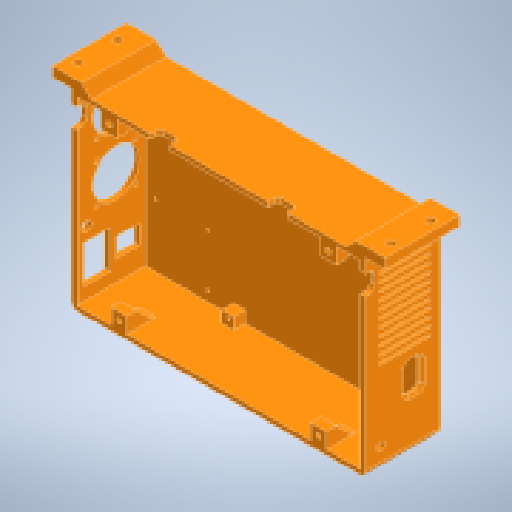
# Autodesk Inventor part: electronic_box
Saved by Autodesk Inventor 2024.1 (Build 281209000, 209)
## iProperties
Created: 2023-10-17
Part Number: electronic_box
Material: Generic
Document SubType Name: Modeling
Designer: l1534
Density: 1 g/cm^3
Appearance: Orange
Author: l1534
Autodesk Inventor part; units mm, degrees
ref_plane "YZ Plane" through (0, 0, 0) normal (1, 0, 0) x (0, 1, 0)
ref_plane "XZ Plane" through (0, 0, 0) normal (0, 1, 0) x (-1, 0, 0)
ref_plane "XY Plane" through (0, 0, 0) normal (0, 0, 1) x (1, 0, 0)
sketch "Sketch1" plane through (0, 0, 0) normal (0, 0, 1) x (1, 0, 0)
  line L0 (-76.6473, 17.8798) -> (73.3527, 17.8798)
  line L1 (73.3527, 17.8798) -> (73.3527, -79.3702)
  line L2 (73.3527, -79.3702) -> (-76.6473, -79.3702)
  line L3 (-76.6473, -79.3702) -> (-76.6473, 17.8798)
  point P0 (0, 0)
  dimension "d0" = 97.25
  dimension "d1" = 150
  constraints: 8 end point, 2 parallel, 1 horizontal, 1 perpendicular
  measures "d0" distance of L0.end L1.end
  measures "d1" distance of L1.end L2.end
extrude "Extrusion1" add sketch "Sketch1" along normal blind 38
sketch "Sketch2" plane through (0, 0, 38) normal (0, 0, 1) x (1, 0, 0)
  line L0 (-74.1473, 15.3798) -> (70.8527, 15.3798)
  line L1 (70.8527, 15.3798) -> (70.8527, -76.8702)
  line L2 (70.8527, -76.8702) -> (-74.1473, -76.8702)
  line L3 (-74.1473, -76.8702) -> (-74.1473, 15.3798)
  line L4 (73.3527, 17.8798) -> (-76.6473, 17.8798) projected
  line L5 (73.3527, -79.3702) -> (73.3527, 17.8798) projected
  line L6 (-76.6473, -79.3702) -> (73.3527, -79.3702) projected
  line L7 (-76.6473, 17.8798) -> (-76.6473, -79.3702) projected
  point P0 (0, 0)
  dimension "d4" = 2.5
  dimension "d5" = 2.5
  dimension "d6" = 2.5
  dimension "d7" = 2.5
  constraints: 8 end point, 2 parallel, 1 horizontal, 1 perpendicular
  measures "d4" distance between parallel lines of L4 L0
  measures "d5" distance between parallel lines of L5 L1
  measures "d6" distance between parallel lines of L6 L2
  measures "d7" distance between parallel lines of L7 L3
extrude "Extrusion2" cut sketch "Sketch2" against normal blind 35 contours L0 L1 L2 L3
sketch "Sketch3" plane through (0, 0, 3) normal (0, 0, 1) x (1, 0, 0)
  line L0 (-74.1473, 15.3798) -> (70.8527, 15.3798) projected
  line L1 (70.8527, 15.3798) -> (64.8527, 15.3798)
  line L2 (64.8527, 15.3798) -> (64.8527, 9.3798)
  line L3 (64.8527, 9.3798) -> (70.8527, 9.3798)
  line L4 (70.8527, 9.3798) -> (70.8527, 15.3798)
  line L5 (70.8527, -76.8702) -> (-74.1473, -76.8702) projected
  line L6 (70.8527, -76.8702) -> (64.8527, -76.8702)
  line L7 (64.8527, -76.8702) -> (64.8527, -70.8702)
  line L8 (64.8527, -70.8702) -> (70.8527, -70.8702)
  line L9 (70.8527, -70.8702) -> (70.8527, -76.8702)
  line L10 (-29.1473, -76.8702) -> (-23.1473, -76.8702)
  line L11 (-23.1473, -76.8702) -> (-23.1473, -70.8702)
  line L12 (-23.1473, -70.8702) -> (-29.1473, -70.8702)
  line L13 (-29.1473, -70.8702) -> (-29.1473, -76.8702)
  line L14 (-29.1473, 15.3798) -> (-23.1473, 15.3798)
  line L15 (-23.1473, 15.3798) -> (-23.1473, 9.3798)
  line L16 (-23.1473, 9.3798) -> (-29.1473, 9.3798)
  line L17 (-29.1473, 9.3798) -> (-29.1473, 15.3798)
  point P0 (0, 0)
  point P1 (64.8527, -73.8702)
  point P2 (-23.1473, -73.8702)
  point P3 (-23.1473, 15.3798)
  point P4 (-29.1473, 15.3798)
  dimension "d10" = 6
  dimension "d11" = 6
  dimension "d12" = 6
  dimension "d13" = 6
  dimension "d14" = 6
  dimension "d15" = 6
  dimension "d16" = 6
  dimension "d17" = 6
  dimension "d18" = 88
  dimension "d19" = 88
  constraints: 32 end point, 8 parallel, 4 horizontal, 4 perpendicular, 2 midpoint, 2 point on line
  measures "d10" distance of L1.end L2.end
  measures "d11" distance of L2.end L3.end
  measures "d12" distance of L7.end L8.end
  measures "d13" distance of L6.end L7.end
  measures "d14" distance of L10.end L11.end
  measures "d15" distance of L11.end L12.end
  measures "d16" distance of L15.end L16.end
  measures "d17" distance of L14.end L15.end
  measures "d18" distance between parallel lines of L2 L15
  measures "d19" distance of point (64.853, -73.87) point (-23.147, -73.87)
extrude "Extrusion3" add sketch "Sketch3" along normal blind 6
sketch "Sketch4" plane through (0, 0, 9) normal (0, 0, 1) x (1, 0, 0)
  circle A0 centre (66.8527, -73.1202) radius 0.9
  line L0 (70.8527, -76.8702) -> (-74.1473, -76.8702) projected
  line L1 (70.8527, 15.3798) -> (70.8527, -76.8702) projected
  point P0 (0, 0)
  dimension "d22" = 1.8
  dimension "d23" = 3.75
  dimension "d24" = 4
  constraints: 1 centre point
  measures "d22" diameter of A0
  measures "d23" distance from line of L0 A0.centre
  measures "d24" distance from line of L1 A0.centre
extrude "Extrusion4" cut sketch "Sketch4" against normal through all
sketch "Sketch5" plane through (0, 0, 9) normal (0, 0, 1) x (1, 0, 0)
  circle A0 centre (66.8527, 11.3798) radius 0.9
  line L0 (64.8527, 9.3798) -> (70.8527, 9.3798) projected
  line L1 (64.8527, 15.3798) -> (64.8527, 9.3798) projected
  point P0 (0, 0)
  dimension "d27" = 1.8
  dimension "d28" = 2
  dimension "d29" = 2
  constraints: 1 centre point
  measures "d27" diameter of A0
  measures "d28" distance from line of L0 A0.centre
  measures "d29" distance from line of L1 A0.centre
extrude "Extrusion5" cut sketch "Sketch5" against normal through all
sketch "Sketch6" plane through (0, 0, 9) normal (0, 0, 1) x (1, 0, 0)
  circle A0 centre (-25.6473, 11.3798) radius 0.9
  circle A1 centre (-25.6473, -73.1202) radius 0.9
  line L0 (-23.1473, 9.3798) -> (-23.1473, 15.3798) projected
  line L1 (-29.1473, 9.3798) -> (-23.1473, 9.3798) projected
  line L2 (-23.1473, -76.8702) -> (-23.1473, -70.8702) projected
  line L3 (-23.1473, -70.8702) -> (-29.1473, -70.8702) projected
  point P0 (0, 0)
  dimension "d32" = 1.8
  dimension "d33" = 1.8
  dimension "d34" = 2.5
  dimension "d35" = 2
  dimension "d36" = 2.5
  dimension "d37" = 2.25
  constraints: 2 centre point
  measures "d32" diameter of A1
  measures "d33" diameter of A0
  measures "d34" distance from line of L0 A0.centre
  measures "d35" distance from line of L1 A0.centre
  measures "d36" distance from line of L2 A1.centre
  measures "d37" distance from line of L3 A1.centre
extrude "Extrusion6" cut sketch "Sketch6" against normal through all
sketch "Sketch7" plane through (70.8527, -76.8702, 38) normal (-1, 0, 0) x (0, 0, 1)
  line L0 (-20.5, 37.5) -> (-28.5, 37.5)
  line L1 (-28.5, 37.5) -> (-28.5, 22.5)
  line L2 (-28.5, 22.5) -> (-20.5, 22.5)
  line L3 (-20.5, 22.5) -> (-20.5, 37.5)
  line L4 (0, 0) -> (-29, 0) projected
  line L5 (-35, 86.25) -> (-35, 6) projected
  point P0 (-38, 76.8702)
  dimension "d40" = 8
  dimension "d41" = 15
  dimension "d42" = 22.5
  dimension "d43" = 6.5
  constraints: 8 end point, 2 parallel, 1 horizontal, 1 perpendicular
  measures "d40" distance of L1.end L2.end
  measures "d41" distance of L2.end L0.start
  measures "d42" distance between parallel lines of L4 L2
  measures "d43" distance between parallel lines of L5 L1
extrude "Extrusion7" cut sketch "Sketch7" against normal through all
fillet "Fillet1" radius 2 4 edges at (72.1027, -39.3702, 9.5) (72.1027, -54.3702, 9.5) (72.1027, -54.3702, 17.5) (72.1027, -39.3702, 17.5)
chamfer "Chamfer1" distance 1.5 angle 45 8 edges at (73.3527, -46.8702, 17.5) (73.3527, -39.956, 16.9142) (73.3527, -39.3702, 13.5) (73.3527, -39.956, 10.0858) (73.3527, -46.8702, 9.5) (73.3527, -53.7844, 10.0858) (73.3527, -54.3702, 13.5) (73.3527, -53.7844, 16.9142)
sketch "Sketch8" plane through (73.3527, -79.3702, 0) normal (1, 0, 0) x (0, 0, -1)
  line L0 (-31, 46) -> (-5, 46)
  line L1 (-5, 46) -> (-5, 47.5)
  line L2 (-5, 47.5) -> (-31, 47.5)
  line L3 (-31, 47.5) -> (-31, 46)
  line L4 (-38, 0) -> (-38, 97.25) projected
  line L5 (0, 0) -> (0, 97.25) projected
  line L6 (0, 0) -> (-38, 0) projected
  line L7 (-31, 50) -> (-5, 50)
  line L8 (-5, 50) -> (-5, 51.5)
  line L9 (-5, 51.5) -> (-31, 51.5)
  line L10 (-31, 51.5) -> (-31, 50)
  line L11 (-31, 54) -> (-5, 54)
  line L12 (-5, 54) -> (-5, 55.5)
  line L13 (-5, 55.5) -> (-31, 55.5)
  line L14 (-31, 55.5) -> (-31, 54)
  line L15 (-31, 58) -> (-5, 58)
  line L16 (-5, 58) -> (-5, 59.5)
  line L17 (-5, 59.5) -> (-31, 59.5)
  line L18 (-31, 59.5) -> (-31, 58)
  line L19 (-31, 62) -> (-5, 62)
  line L20 (-5, 62) -> (-5, 63.5)
  line L21 (-5, 63.5) -> (-31, 63.5)
  line L22 (-31, 63.5) -> (-31, 62)
  line L23 (-31, 66) -> (-5, 66)
  line L24 (-5, 66) -> (-5, 67.5)
  line L25 (-5, 67.5) -> (-31, 67.5)
  line L26 (-31, 67.5) -> (-31, 66)
  line L27 (-31, 70) -> (-5, 70)
  line L28 (-5, 70) -> (-5, 71.5)
  line L29 (-5, 71.5) -> (-31, 71.5)
  line L30 (-31, 71.5) -> (-31, 70)
  line L31 (-31, 74) -> (-5, 74)
  line L32 (-5, 74) -> (-5, 75.5)
  line L33 (-5, 75.5) -> (-31, 75.5)
  line L34 (-31, 75.5) -> (-31, 74)
  line L35 (-31, 78) -> (-5, 78)
  line L36 (-5, 78) -> (-5, 79.5)
  line L37 (-5, 79.5) -> (-31, 79.5)
  line L38 (-31, 79.5) -> (-31, 78)
  line L39 (-31, 82) -> (-5, 82)
  line L40 (-5, 82) -> (-5, 83.5)
  line L41 (-5, 83.5) -> (-31, 83.5)
  line L42 (-31, 83.5) -> (-31, 82)
  line L43 (-31, 86) -> (-5, 86)
  line L44 (-5, 86) -> (-5, 87.5)
  line L45 (-5, 87.5) -> (-31, 87.5)
  line L46 (-31, 87.5) -> (-31, 86)
  point P0 (0, 79.3702)
  dimension "d50" = 1.5
  dimension "d51" = 7
  dimension "d52" = 5
  dimension "d53" = 46
  dimension "d56" = 4
  constraints: 88 end point, 2 parallel, 1 horizontal, 1 perpendicular, 1 vertical, 80 other
  measures "d50" distance of L2.end L0.start
  measures "d51" distance between parallel lines of L4 L3
  measures "d52" distance between parallel lines of L5 L1
  measures "d53" distance between parallel lines of L6 L0
  measures "d56" distance of L0.start L7.start
extrude "Extrusion8" cut sketch "Sketch8" against normal up to surface (2.5 mm away)
fillet "Fillet2" radius 0.75 44 edges at (72.1027, -33.3702, 31) (72.1027, -31.8702, 31) (72.1027, -29.3702, 31) (72.1027, -27.8702, 31) (72.1027, -25.3702, 31) (72.1027, -21.3702, 31) (72.1027, -17.3702, 31) (72.1027, -13.3702, 31) (72.1027, -9.3702, 31) (72.1027, -5.3702, 31) (72.1027, -1.3702, 31) (72.1027, 2.6298, 31) (72.1027, 6.6298, 31) (72.1027, -33.3702, 5) (72.1027, -29.3702, 5) (72.1027, -25.3702, 5) (72.1027, -21.3702, 5) (72.1027, -17.3702, 5) (72.1027, -13.3702, 5) (72.1027, -9.3702, 5) (72.1027, -5.3702, 5) (72.1027, -1.3702, 5) (72.1027, 2.6298, 5) (72.1027, 6.6298, 5) (72.1027, 8.1298, 5) (72.1027, 4.1298, 5) (72.1027, 0.1298, 5) (72.1027, -3.8702, 5) (72.1027, -7.8702, 5) (72.1027, -11.8702, 5) (72.1027, -15.8702, 5) (72.1027, -19.8702, 5) (72.1027, -23.8702, 5) (72.1027, -27.8702, 5) (72.1027, -31.8702, 5) (72.1027, 8.1298, 31) (72.1027, 4.1298, 31) (72.1027, 0.1298, 31) (72.1027, -3.8702, 31) (72.1027, -7.8702, 31) (72.1027, -11.8702, 31) (72.1027, -15.8702, 31) (72.1027, -19.8702, 31) (72.1027, -23.8702, 31)
sketch "Sketch10" plane through (-76.6473, -79.3702, 0) normal (-1, 0, 0) x (0, 0, 1)
  circle A0 centre (18, 81.25) radius 12
  line L0 (0, 97.25) -> (38, 97.25) projected
  line L1 (38, 97.25) -> (38, 0) projected
  circle A1 centre (18, 51.25) radius 12
  point P0 (0, 79.3702)
  dimension "d64" = 24
  dimension "d66" = 16
  dimension "d67" = 20
  dimension "d93" = 30
  constraints: 2 centre point, 1 vertical, 2 other
  measures "d64" diameter of A0
  measures "d66" distance from line of L0 A0.centre
  measures "d67" distance from line of L1 A0.centre
  measures "d93" distance of A0.centre A1.centre
extrude "Extrusion9" cut sketch "Sketch10" against normal up to surface (2.5 mm away)
sketch "Sketch11" plane through (-76.6473, -79.3702, 0) normal (-1, 0, 0) x (0, 0, 1)
  circle A0 centre (28, 91.25) radius 1.1
  circle A1 centre (28, 71.25) radius 1.1
  circle A2 centre (8, 71.25) radius 1.1
  line L0 (30.25, 87.5) -> (5.75, 87.5) projected
  circle A3 centre (18, 81.25) radius 12 projected
  circle A4 centre (8, 91.25) radius 1.1
  line L1 (35.0639, 55.5) -> (35.0639, 30.8182)
  circle A5 centre (28, 61.25) radius 1.1
  circle A6 centre (8, 61.25) radius 1.1
  circle A7 centre (8, 41.25) radius 1.1
  circle A8 centre (28, 41.25) radius 1.1
  point P0 (0, 79.3702)
  dimension "d72" = 2.2
  dimension "d73" = 2.2
  dimension "d75" = 2.2
  dimension "d76" = 10
  dimension "d77" = 10
  dimension "d79" = 10
  dimension "d80" = 10
  dimension "d81" = 10
  dimension "d82" = 10
  dimension "d83" = 2.2
  dimension "d84" = 10
  dimension "d85" = 10
  dimension "d100" = 30
  constraints: 8 centre point, 2 end point, 2 vertical, 8 other
  measures "d72" diameter of A0
  measures "d73" diameter of A1
  measures "d75" diameter of A2
  measures "d76" horizontal distance of A3.centre A0.centre
  measures "d77" horizontal distance of A3.centre A1.centre
  measures "d79" horizontal distance of A3.centre A2.centre
  measures "d80" horizontal distance of A3.centre A2.centre
  measures "d81" horizontal distance of A3.centre A1.centre
  measures "d82" horizontal distance of A3.centre A0.centre
  measures "d83" diameter of A4
  measures "d84" horizontal distance of A3.centre A4.centre
  measures "d85" horizontal distance of A3.centre A4.centre
  measures "d100" distance of A0.centre A5.centre
extrude "Extrusion10" cut sketch "Sketch11" against normal up to surface (2.5 mm away) contours A0 | A1 | A2 | A4 | A5 | A6 | A7 | A8
chamfer "Chamfer2" distance 1.5 angle 45 1 edges at (-1.6473, -79.3702, 0)
sketch "Sketch12" plane through (-76.6473, -79.3702, 38) normal (-1, 0, 0) x (0, 0, 1)
  line L0 (-3.8, 28.5) -> (-17, 28.5)
  line L1 (-17, 28.5) -> (-17, 9)
  line L2 (-17, 9) -> (-3.8, 9)
  line L3 (-3.8, 9) -> (-3.8, 28.5)
  line L4 (-38, 95.75) -> (-38, 1.5) projected
  line L5 (-36.5, 0) -> (0, 0) projected
  point P0 (-38, 79.3702)
  dimension "d105" = 13.2
  dimension "d106" = 19.5
  dimension "d107" = 21
  dimension "d108" = 9
  constraints: 8 end point, 2 parallel, 1 horizontal, 1 perpendicular
  measures "d105" distance of L1.end L2.end
  measures "d106" distance of L0.end L1.end
  measures "d107" distance between parallel lines of L4 L1
  measures "d108" distance between parallel lines of L5 L2
extrude "Extrusion11" cut sketch "Sketch12" against normal up to surface (2.5 mm away)
sketch "Sketch13" plane through (-76.6473, -79.3702, 38) normal (-1, 0, 0) x (0, 0, 1)
  line L0 (0, 97.25) -> (0, 0) projected
  line L1 (0, 90.25) -> (-5, 90.25)
  line L2 (-5, 90.25) -> (-5, 80.25)
  line L3 (-5, 80.25) -> (0, 80.25)
  line L4 (0, 80.25) -> (0, 90.25)
  line L5 (-38, 97.25) -> (0, 97.25) projected
  point P0 (-38, 79.3702)
  point P1 (-36.5, 97.25)
  point P2 (0, 80.25)
  dimension "d111" = 5
  dimension "d112" = 10
  dimension "d113" = 7
  constraints: 8 end point, 2 parallel, 1 horizontal, 1 perpendicular, 1 point on line
  measures "d111" distance of L2.end L3.end
  measures "d112" distance of L1.end L2.end
  measures "d113" distance between parallel lines of L5 L1
extrude "Extrusion12" cut sketch "Sketch13" against normal through all
fillet "Fillet3" radius 3 4 edges at (-75.3973, 10.8798, 33) (-75.3973, 0.8798, 33) (72.1027, 10.8798, 33) (72.1027, 0.8798, 33)
fillet "Fillet4" radius 3 2 edges at (73.3527, -79.3702, 19.75) (-76.6473, -79.3702, 19.75)
sketch "Sketch14" plane through (-76.6473, 17.8798, 1.5) normal (-1, 0, 0) x (0, 0, 1)
  line L0 (16.5, -74.25) -> (4.5, -74.25)
  line L1 (4.5, -74.25) -> (4.5, -84.25)
  line L2 (4.5, -84.25) -> (16.5, -84.25)
  line L3 (16.5, -84.25) -> (16.5, -74.25)
  line L4 (-1.5, -1.5) -> (-1.5, -95.75) projected
  line L5 (0, -97.25) -> (36.5, -97.25) projected
  point P0 (-1.5, -17.8798)
  dimension "d118" = 12
  dimension "d119" = 10
  dimension "d120" = 6
  dimension "d121" = 13
  constraints: 8 end point, 2 parallel, 1 horizontal, 1 perpendicular
  measures "d118" distance of L1.end L2.end
  measures "d119" distance of L2.end L0.start
  measures "d120" distance between parallel lines of L4 L1
  measures "d121" distance between parallel lines of L5 L2
extrude "Extrusion13" cut sketch "Sketch14" against normal up to surface (2.5 mm away)
sketch "Sketch15" plane through (73.3527, 17.8798, 38) normal (1, 0, 0) x (0, 0, -1)
  circle A0 centre (8, -87.25) radius 2
  line L0 (0, -94.25) -> (0, -17) projected
  line L1 (0, -97.25) -> (36.5, -97.25) projected
  point P0 (38, -17.8798)
  dimension "d124" = 4
  dimension "d125" = 8
  dimension "d126" = 10
  constraints: 1 centre point
  measures "d124" diameter of A0
  measures "d125" distance from line of L0 A0.centre
  measures "d126" distance from line of L1 A0.centre
extrude "Extrusion14" cut sketch "Sketch15" against normal up to surface (2.5 mm away)
sketch "Sketch16" plane through (-76.6473, 17.8798, 1.5) normal (-1, 0, 0) x (0, 0, 1)
  circle A0 centre (31.5, -62.25) radius 2.5
  line L0 (36.5, -17) -> (36.5, -94.25) projected
  line L1 (0, -97.25) -> (36.5, -97.25) projected
  point P0 (-1.5, -17.8798)
  dimension "d129" = 5
  dimension "d130" = 5
  dimension "d131" = 35
  constraints: 1 centre point
  measures "d129" diameter of A0
  measures "d130" distance from line of L0 A0.centre
  measures "d131" distance from line of L1 A0.centre
extrude "Extrusion15" cut sketch "Sketch16" against normal up to surface (2.5 mm away)
sketch "Sketch17" plane through (0, 0, 3) normal (0, 0, 1) x (1, 0, 0)
  circle A0 centre (-69.1473, -44.8702) radius 0.8
  circle A1 centre (-42.1473, -44.8702) radius 0.8
  circle A2 centre (-42.1473, -71.8702) radius 0.8
  line L0 (-74.1473, -76.8702) -> (-74.1473, 0.8798) projected
  line L1 (70.8527, -76.8702) -> (-74.1473, -76.8702) projected
  point P0 (0, 0)
  dimension "d134" = 1.6
  dimension "d135" = 1.6
  dimension "d136" = 1.6
  dimension "d137" = 5
  dimension "d138" = 32
  dimension "d139" = 32
  dimension "d140" = 32
  dimension "d141" = 5
  dimension "d142" = 32
  constraints: 3 centre point
  measures "d134" diameter of A0
  measures "d135" diameter of A1
  measures "d136" diameter of A2
  measures "d137" distance from line of L0 A0.centre
  measures "d138" distance from line of L1 A0.centre
  measures "d139" distance from line of L1 A1.centre
  measures "d140" distance from line of L0 A1.centre
  measures "d141" distance from line of L1 A2.centre
  measures "d142" distance from line of L0 A2.centre
extrude "Extrusion16" cut sketch "Sketch17" against normal up to surface (3 mm away)
sketch "Sketch18" plane through (-76.6473, 17.8798, 0) normal (0, 1, 0) x (1, 0, 0)
  line L0 (145, -38) -> (160, -38)
  line L1 (160, -38) -> (160, 0)
  line L2 (160, 0) -> (145, 0)
  line L3 (145, 0) -> (145, -38)
  line L4 (150, -38) -> (0, -38) projected
  line L5 (5, -38) -> (-10, -38)
  line L6 (-10, -38) -> (-10, 0)
  line L7 (-10, 0) -> (5, 0)
  line L8 (5, 0) -> (5, -38)
  line L9 (150, 0) -> (150, -38) projected
  line L10 (0, 0) -> (0, -38) projected
  point P0 (76.6473, 0)
  dimension "d145" = 15
  dimension "d146" = 15
  dimension "d147" = 38
  dimension "d148" = 38
  dimension "d149" = 5
  dimension "d150" = 5
  constraints: 16 end point, 4 parallel, 2 horizontal, 2 perpendicular, 1 point on line
  measures "d145" distance of L5.start L5.end
  measures "d146" distance of L0.start L0.end
  measures "d147" distance of L2.end L0.start
  measures "d148" distance of L5.end L6.end
  measures "d149" distance between parallel lines of L9 L3
  measures "d150" distance between parallel lines of L10 L8
extrude "Extrusion17" add sketch "Sketch18" along normal blind 5
chamfer "Chamfer3" distance 5 angle 45 2 edges at (-71.6473, 17.8798, 19) (68.3527, 17.8798, 19)
sketch "Sketch19" plane through (-76.6473, 17.8798, 0) normal (0, -1, 0) x (1, 0, 0)
  circle A0 centre (155, 30) radius 2.1
  circle A1 centre (155, 10) radius 2.1
  circle A2 centre (-5, 30) radius 2.1
  circle A3 centre (-5, 10) radius 2.1
  line L0 (-10, 38) -> (0, 38) projected
  line L1 (-10, 0) -> (-10, 38) projected
  line L2 (0, 0) -> (-10, 0) projected
  line L3 (160, 38) -> (160, 0) projected
  line L4 (150, 38) -> (160, 38) projected
  line L5 (160, 0) -> (150, 0) projected
  point P0 (76.6473, 0)
  dimension "d156" = 4.2
  dimension "d157" = 4.2
  dimension "d158" = 4.2
  dimension "d159" = 4.2
  dimension "d160" = 8
  dimension "d161" = 5
  dimension "d162" = 10
  dimension "d163" = 5
  dimension "d164" = 5
  dimension "d165" = 8
  dimension "d166" = 5
  dimension "d167" = 10
  constraints: 4 centre point
  measures "d156" diameter of A1
  measures "d157" diameter of A0
  measures "d158" diameter of A3
  measures "d159" diameter of A2
  measures "d160" distance from line of L0 A2.centre
  measures "d161" distance from line of L1 A2.centre
  measures "d162" distance from line of L2 A3.centre
  measures "d163" distance from line of L1 A3.centre
  measures "d164" distance from line of L3 A0.centre
  measures "d165" distance from line of L4 A0.centre
  measures "d166" distance from line of L3 A1.centre
  measures "d167" distance from line of L5 A1.centre
extrude "Extrusion18" cut sketch "Sketch19" against normal up to surface (5 mm away)
sketch "Sketch20" plane through (0, 0, 38) normal (0, 0, 1) x (1, 0, 0)
  line L0 (63.3527, 17.8798) -> (-66.6473, 17.8798) projected
  line L1 (-61.6473, 17.8798) -> (-53.6473, 17.8798)
  line L2 (-53.6473, 17.8798) -> (-53.6473, 7.3798)
  line L3 (-53.6473, 7.3798) -> (-61.6473, 7.3798)
  line L4 (-61.6473, 7.3798) -> (-61.6473, 17.8798)
  line L5 (50.3527, 17.8798) -> (58.3527, 17.8798)
  line L6 (58.3527, 17.8798) -> (58.3527, 7.3798)
  line L7 (58.3527, 7.3798) -> (50.3527, 7.3798)
  line L8 (50.3527, 7.3798) -> (50.3527, 17.8798)
  line L9 (70.3527, -79.3702) -> (-73.6473, -79.3702) projected
  line L10 (45.3527, -79.3702) -> (53.3527, -79.3702)
  line L11 (53.3527, -79.3702) -> (53.3527, -68.8702)
  line L12 (53.3527, -68.8702) -> (45.3527, -68.8702)
  line L13 (45.3527, -68.8702) -> (45.3527, -79.3702)
  line L14 (-56.6473, -79.3702) -> (-48.6473, -79.3702)
  line L15 (-48.6473, -79.3702) -> (-48.6473, -68.8702)
  line L16 (-48.6473, -68.8702) -> (-56.6473, -68.8702)
  line L17 (-56.6473, -68.8702) -> (-56.6473, -79.3702)
  line L18 (73.3527, 10.8798) -> (73.3527, 17.8798) projected
  line L19 (-76.6473, 17.8798) -> (-76.6473, 10.8798) projected
  line L20 (-76.6473, 0.8798) -> (-76.6473, -76.3702) projected
  line L21 (73.3527, -76.3702) -> (73.3527, 0.8798) projected
  point P0 (0, 0)
  dimension "d170" = 8
  dimension "d171" = 10.5
  dimension "d172" = 8
  dimension "d173" = 10.5
  dimension "d174" = 10.5
  dimension "d175" = 8
  dimension "d176" = 8
  dimension "d177" = 10.5
  dimension "d178" = 15
  dimension "d179" = 15
  dimension "d180" = 20
  dimension "d181" = 20
  constraints: 32 end point, 8 parallel, 5 point on line, 4 horizontal, 4 perpendicular
  measures "d170" distance of L15.end L16.end
  measures "d171" distance of L16.end L14.start
  measures "d172" distance of L11.end L12.end
  measures "d173" distance of L10.end L11.end
  measures "d174" distance of L5.end L6.end
  measures "d175" distance of L6.end L7.end
  measures "d176" distance of L2.end L3.end
  measures "d177" distance of L1.end L2.end
  measures "d178" distance between parallel lines of L18 L6
  measures "d179" distance between parallel lines of L19 L4
  measures "d180" distance between parallel lines of L20 L17
  measures "d181" distance between parallel lines of L21 L11
extrude "Extrusion19" add sketch "Sketch20" against normal blind 5
chamfer "Chamfer4" distance 8 angle 45 4 edges at (-57.6473, 15.3798, 33) (54.3527, 15.3798, 33) (-52.6473, -76.8702, 33) (49.3527, -76.8702, 33)
sketch "Sketch21" plane through (0, 0, 38) normal (0, 0, 1) x (1, 0, 0)
  circle A0 centre (-57.6473, 11.3798) radius 1.3
  circle A1 centre (54.3527, 11.3798) radius 1.3
  circle A2 centre (49.3527, -72.8702) radius 1.3
  circle A3 centre (-52.6473, -72.8702) radius 1.3
  line L0 (-48.6473, -68.8702) -> (-56.6473, -68.8702) projected
  line L1 (-48.6473, -76.8702) -> (-48.6473, -68.8702) projected
  line L2 (53.3527, -76.8702) -> (53.3527, -68.8702) projected
  line L3 (53.3527, -68.8702) -> (45.3527, -68.8702) projected
  line L4 (58.3527, 7.3798) -> (58.3527, 15.3798) projected
  line L5 (50.3527, 7.3798) -> (58.3527, 7.3798) projected
  line L6 (-61.6473, 7.3798) -> (-53.6473, 7.3798) projected
  line L7 (-53.6473, 7.3798) -> (-53.6473, 15.3798) projected
  point P0 (0, 0)
  dimension "d187" = 2.6
  dimension "d188" = 2.6
  dimension "d189" = 2.6
  dimension "d190" = 2.6
  dimension "d191" = 4
  dimension "d192" = 4
  dimension "d193" = 4
  dimension "d194" = 4
  dimension "d195" = 4
  dimension "d196" = 4
  dimension "d197" = 4
  dimension "d198" = 4
  constraints: 4 centre point
  measures "d187" diameter of A0
  measures "d188" diameter of A1
  measures "d189" diameter of A2
  measures "d190" diameter of A3
  measures "d191" distance from line of L0 A3.centre
  measures "d192" distance from line of L1 A3.centre
  measures "d193" distance from line of L2 A2.centre
  measures "d194" distance from line of L3 A2.centre
  measures "d195" distance from line of L4 A1.centre
  measures "d196" distance from line of L5 A1.centre
  measures "d197" distance from line of L6 A0.centre
  measures "d198" distance from line of L7 A0.centre
extrude "Extrusion20" cut sketch "Sketch21" against normal up to surface (35 mm away)
fillet "Fillet5" radius 5 4 edges at (-52.6473, -76.8702, 25.0001) (49.3527, -76.8702, 25.0001) (-57.6473, 15.3798, 25.0001) (54.3527, 15.3798, 25.0001)
sketch "Sketch22" plane through (0, 0, 38) normal (0, 0, 1) x (1, 0, 0)
  line L0 (63.3527, 17.8798) -> (-66.6473, 17.8798) projected
  line L1 (-23.1473, 15.3798) -> (64.8527, 15.3798) projected
  line L2 (-36.6473, 17.8798) -> (-26.6473, 17.8798)
  line L3 (-26.6473, 17.8798) -> (-26.6473, 15.3798)
  line L4 (-26.6473, 15.3798) -> (-36.6473, 15.3798)
  line L5 (-36.6473, 15.3798) -> (-36.6473, 17.8798)
  line L6 (23.3527, 17.8798) -> (33.3527, 17.8798)
  line L7 (33.3527, 17.8798) -> (33.3527, 15.3798)
  line L8 (33.3527, 15.3798) -> (23.3527, 15.3798)
  line L9 (23.3527, 15.3798) -> (23.3527, 17.8798)
  line L10 (-76.6473, 17.8798) -> (-76.6473, 10.8798) projected
  line L11 (73.3527, 10.8798) -> (73.3527, 17.8798) projected
  point P0 (0, 0)
  dimension "d202" = 10
  dimension "d203" = 10
  dimension "d204" = 40
  dimension "d205" = 40
  constraints: 16 end point, 4 parallel, 4 point on line, 2 horizontal, 2 perpendicular
  measures "d202" distance between parallel lines of L3 L5
  measures "d203" distance between parallel lines of L7 L9
  measures "d204" distance between parallel lines of L10 L5
  measures "d205" distance between parallel lines of L11 L7
extrude "Extrusion21" cut sketch "Sketch22" against normal blind 5
fillet "Fillet6" radius 2 4 edges at (-26.6473, 16.6298, 33) (33.3527, 16.6298, 33) (23.3527, 16.6298, 33) (-36.6473, 16.6298, 33)
body "Solid1"
